Autodesk Fusion 360 part; units mm, degrees
(part 2 of 2)
sketch "Sketch2" plane through (0, 0, 25) normal (0, 0, 1) x (-1, 0, 0)
  spline S0 degree 3 poles (-93.3378, -102.7633) (-92.6534, -103.4892) (-92.135, -104.0698) (-92.1764, -104.0698) knots -1 -1 -1 -1 0 0 0 0
  spline S1 degree 3 poles (-92.1764, -104.0698) (-92.4046, -104.0698) (-94.6651, -102.2863) (-95.5154, -101.436) knots -1 -1 -1 -1 0 0 0 0
  spline S2 degree 3 poles (-95.5154, -101.436) (-96.0131, -100.9383) (-96.5938, -100.4406) (-96.8219, -100.3161) knots -1 -1 -1 -1 0 0 0 0
  spline S3 degree 3 poles (-96.8219, -100.3161) (-97.0293, -100.2125) (-97.1537, -100.0258) (-97.0915, -99.9014) knots -1 -1 -1 -1 0 0 0 0
  spline S4 degree 3 poles (-97.0915, -99.9014) (-97.0085, -99.7977) (-97.1537, -99.7147) (-97.3818, -99.7147) knots -1 -1 -1 -1 0 0 0 0
  spline S5 degree 3 poles (-97.3818, -99.7147) (-97.6307, -99.7147) (-97.921, -99.5281) (-98.0662, -99.3) knots -1 -1 -1 -1 0 0 0 0
  spline S6 degree 3 poles (-98.0662, -99.3) (-98.2114, -99.0718) (-98.4395, -98.8852) (-98.5847, -98.8852) knots -1 -1 -1 -1 0 0 0 0
  spline S7 degree 3 poles (-98.5847, -98.8852) (-98.7299, -98.8852) (-98.9165, -98.7608) (-98.9995, -98.5948) knots -1 -1 -1 -1 0 0 0 0
  spline S8 degree 3 poles (-98.9995, -98.5948) (-99.0824, -98.4289) (-99.4557, -97.9727) (-99.8083, -97.5786) knots -1 -1 -1 -1 0 0 0 0
  spline S9 degree 3 poles (-99.8083, -97.5786) (-101.0111, -96.2721) (-104.433, -91.6267) (-105.1588, -90.3201) knots -1 -1 -1 -1 0 0 0 0
  spline S10 degree 3 poles (-105.1588, -90.3201) (-106.258, -88.3707) (-108.1452, -83.663) (-108.7051, -81.5269) knots -1 -1 -1 -1 0 0 0 0
  spline S11 degree 3 poles (-108.7051, -81.5269) (-109.8043, -77.3377) (-110.2191, -72.4434) (-109.8665, -67.9639) knots -1 -1 -1 -1 0 0 0 0
  spline S12 degree 3 poles (-109.8665, -67.9639) (-109.5347, -63.7539) (-107.9171, -58.1545) (-106.1128, -54.8156) knots -1 -1 -1 -1 0 0 0 0
  spline S13 degree 3 poles (-106.1128, -54.8156) (-105.7395, -54.1312) (-105.2211, -53.2187) (-104.9929, -52.7624) knots -1 -1 -1 -1 0 0 0 0
  spline S14 degree 3 poles (-104.9929, -52.7624) (-104.7441, -52.3269) (-104.433, -51.9122) (-104.3086, -51.8707) knots -1 -1 -1 -1 0 0 0 0
  spline S15 degree 3 poles (-104.3086, -51.8707) (-104.1634, -51.8085) (-104.0389, -51.6011) (-104.0182, -51.4144) knots -1 -1 -1 -1 0 0 0 0
  spline S16 degree 3 poles (-104.0182, -51.4144) (-104.0182, -51.2278) (-103.956, -51.1863) (-103.8938, -51.3315) knots -1 -1 -1 -1 0 0 0 0
  spline S17 degree 3 poles (-103.8938, -51.3315) (-103.7693, -51.6633) (-103.1679, -51.0619) (-101.8407, -49.3198) knots -1 -1 -1 -1 0 0 0 0
  spline S18 degree 3 poles (-101.8407, -49.3198) (-99.6424, -46.3749) (-96.9256, -43.7411) (-93.6904, -41.3769) knots -1 -1 -1 -1 0 0 0 0
  spline S19 degree 3 poles (-93.6904, -41.3769) (-91.0151, -39.4275) (-86.5563, -36.9803) (-86.0171, -37.1877) knots -1 -1 -1 -1 0 0 0 0
  spline S20 degree 3 poles (-86.0171, -37.1877) (-85.8512, -37.2499) (-85.7682, -37.2499) (-85.8512, -37.167) knots -1 -1 -1 -1 0 0 0 0
  spline S21 degree 3 poles (-85.8512, -37.167) (-86.0585, -36.9596) (-83.3003, -35.7982) (-82.9478, -35.9434) knots -1 -1 -1 -1 0 0 0 0
  spline S22 degree 3 poles (-82.9478, -35.9434) (-82.7818, -35.9849) (-82.6989, -35.9641) (-82.7611, -35.8605) knots -1 -1 -1 -1 0 0 0 0
  spline S23 degree 3 poles (-82.7611, -35.8605) (-82.8233, -35.7568) (-82.6367, -35.6116) (-82.3049, -35.5494) knots -1 -1 -1 -1 0 0 0 0
  spline S24 degree 3 poles (-82.3049, -35.5494) (-81.9938, -35.4664) (-81.1435, -35.2383) (-80.3969, -35.0102) knots -1 -1 -1 -1 0 0 0 0
  spline S25 degree 3 poles (-80.3969, -35.0102) (-77.7009, -34.2428) (-77.2031, -34.1391) (-73.6983, -33.7451) knots -1 -1 -1 -1 0 0 0 0
  spline S26 degree 3 poles (-73.6983, -33.7451) (-69.8824, -33.3303) (-66.7924, -33.2474) (-66.2946, -33.5585) knots -1 -1 -1 -1 0 0 0 0
  spline S27 degree 3 poles (-66.2946, -33.5585) (-65.9628, -33.7659) (-66.1702, -33.8695) (-68.6796, -34.6991) knots -1 -1 -1 -1 0 0 0 0
  spline S28 degree 3 poles (-68.6796, -34.6991) (-70.8364, -35.4042) (-71.9355, -35.9641) (-74.4656, -37.6647) knots -1 -1 -1 -1 0 0 0 0
  spline S29 degree 3 poles (-74.4656, -37.6647) (-80.5421, -41.7502) (-87.054, -48.0963) (-90.2063, -53.0113) knots -1 -1 -1 -1 0 0 0 0
  spline S30 degree 3 poles (-90.2063, -53.0113) (-92.1142, -55.9562) (-93.4622, -59.1292) (-93.4622, -60.7053) knots -1 -1 -1 -1 0 0 0 0
  line L0 (-93.4622, -60.7053) -> (-93.483, -61.4519)
  line L1 (-93.483, -61.4519) -> (-94.0014, -60.8298)
  spline S31 degree 3 poles (-94.0014, -60.8298) (-95.6191, -58.8596) (-95.5154, -54.9815) (-93.6904, -49.4235) knots -1 -1 -1 -1 0 0 0 0
  spline S32 degree 3 poles (-93.6904, -49.4235) (-93.3585, -48.4073) (-93.1097, -47.5156) (-93.1512, -47.4741) knots -1 -1 -1 -1 0 0 0 0
  spline S33 degree 3 poles (-93.1512, -47.4741) (-93.3585, -47.2874) (-96.5108, -49.942) (-97.8588, -51.4144) knots -1 -1 -1 -1 0 0 0 0
  spline S34 degree 3 poles (-97.8588, -51.4144) (-101.8614, -55.811) (-103.6242, -59.3988) (-103.6242, -63.1525) knots -1 -1 -1 -1 0 0 0 0
  spline S35 degree 3 poles (-103.6242, -63.1525) (-103.6242, -66.1389) (-102.608, -69.0215) (-99.912, -73.584) knots -1 -1 -1 -1 0 0 0 0
  spline S36 degree 3 poles (-99.912, -73.584) (-97.8588, -77.0889) (-97.3404, -80.5522) (-98.2114, -84.9488) knots -1 -1 -1 -1 0 0 0 0
  spline S37 degree 3 poles (-98.2114, -84.9488) (-98.4603, -86.1309) (-98.7091, -87.9974) (-98.7713, -89.0965) knots -1 -1 -1 -1 0 0 0 0
  spline S38 degree 3 poles (-98.7713, -89.0965) (-99.0617, -93.8042) (-96.9878, -99.0511) (-93.3378, -102.7633) knots -1 -1 -1 -1 0 0 0 0
  spline S39 degree 3 poles (-53.9551, -98.2838) (-55.4691, -98.5119) (-56.6926, -98.346) (-58.1236, -97.6616) knots -1 -1 -1 -1 0 0 0 0
  spline S40 degree 3 poles (-58.1236, -97.6616) (-60.7989, -96.4173) (-63.1216, -93.1198) (-63.7023, -89.7394) knots -1 -1 -1 -1 0 0 0 0
  spline S41 degree 3 poles (-63.7023, -89.7394) (-63.8889, -88.7232) (-63.4327, -85.6954) (-62.9557, -84.7) knots -1 -1 -1 -1 0 0 0 0
  spline S42 degree 3 poles (-62.9557, -84.7) (-62.6031, -83.9534) (-62.5617, -83.5801) (-62.6861, -81.5477) knots -1 -1 -1 -1 0 0 0 0
  spline S43 degree 3 poles (-62.6861, -81.5477) (-62.8313, -78.9968) (-62.7691, -78.7272) (-61.5455, -77.5036) knots -1 -1 -1 -1 0 0 0 0
  spline S44 degree 3 poles (-61.5455, -77.5036) (-61.1307, -77.0889) (-60.5915, -76.4667) (-60.3219, -76.1142) knots -1 -1 -1 -1 0 0 0 0
  spline S45 degree 3 poles (-60.3219, -76.1142) (-59.5753, -75.098) (-57.5014, -74.7247) (-56.0497, -75.3261) knots -1 -1 -1 -1 0 0 0 0
  spline S46 degree 3 poles (-56.0497, -75.3261) (-55.6764, -75.4713) (-54.8884, -76.0312) (-54.287, -76.5704) knots -1 -1 -1 -1 0 0 0 0
  spline S47 degree 3 poles (-54.287, -76.5704) (-53.7063, -77.0889) (-52.856, -77.711) (-52.4412, -77.9184) knots -1 -1 -1 -1 0 0 0 0
  spline S48 degree 3 poles (-52.4412, -77.9184) (-51.1139, -78.6028) (-50.16, -79.7642) (-49.7037, -81.2366) knots -1 -1 -1 -1 0 0 0 0
  spline S49 degree 3 poles (-49.7037, -81.2366) (-49.206, -82.8127) (-49.206, -82.792) (-49.6, -82.6261) knots -1 -1 -1 -1 0 0 0 0
  spline S50 degree 3 poles (-49.6, -82.6261) (-49.7867, -82.5639) (-49.9111, -82.6261) (-49.9111, -82.8335) knots -1 -1 -1 -1 0 0 0 0
  spline S51 degree 3 poles (-49.9111, -82.8335) (-49.9111, -82.9994) (-49.9941, -83.0823) (-50.1185, -83.0201) knots -1 -1 -1 -1 0 0 0 0
  spline S52 degree 3 poles (-50.1185, -83.0201) (-50.2222, -82.9579) (-50.2637, -83.0201) (-50.2222, -83.1653) knots -1 -1 -1 -1 0 0 0 0
  spline S53 degree 3 poles (-50.2222, -83.1653) (-50.0977, -83.4764) (-51.2798, -84.7207) (-51.7776, -84.8244) knots -1 -1 -1 -1 0 0 0 0
  spline S54 degree 3 poles (-51.7776, -84.8244) (-52.5034, -84.9696) (-53.25, -86.3176) (-53.7685, -88.3914) knots -1 -1 -1 -1 0 0 0 0
  line L2 (-53.7685, -88.3914) -> (-54.1003, -89.7602)
  line L3 (-54.1003, -89.7602) -> (-54.9506, -89.0758)
  spline S55 degree 3 poles (-54.9506, -89.0758) (-56.3193, -87.9974) (-56.7548, -87.8315) (-58.6835, -87.7278) knots -1 -1 -1 -1 0 0 0 0
  spline S56 degree 3 poles (-58.6835, -87.7278) (-59.679, -87.6863) (-60.4878, -87.5619) (-60.4878, -87.4582) knots -1 -1 -1 -1 0 0 0 0
  spline S57 degree 3 poles (-60.4878, -87.4582) (-60.4878, -87.3545) (-60.633, -87.2715) (-60.8196, -87.2715) knots -1 -1 -1 -1 0 0 0 0
  spline S58 degree 3 poles (-60.8196, -87.2715) (-61.0063, -87.2715) (-61.11, -87.4167) (-61.0685, -87.6241) knots -1 -1 -1 -1 0 0 0 0
  spline S59 degree 3 poles (-61.0685, -87.6241) (-61.027, -87.8522) (-60.6537, -88.0389) (-59.8656, -88.184) knots -1 -1 -1 -1 0 0 0 0
  spline S60 degree 3 poles (-59.8656, -88.184) (-58.0821, -88.5573) (-56.7963, -89.3039) (-55.1165, -90.9423) knots -1 -1 -1 -1 0 0 0 0
  spline S61 degree 3 poles (-55.1165, -90.9423) (-54.287, -91.7718) (-53.5611, -92.4562) (-53.5196, -92.4562) knots -1 -1 -1 -1 0 0 0 0
  spline S62 degree 3 poles (-53.5196, -92.4562) (-53.4781, -92.4562) (-53.4367, -92.3318) (-53.4367, -92.1659) knots -1 -1 -1 -1 0 0 0 0
  spline S63 degree 3 poles (-53.4367, -92.1659) (-53.4367, -92.0207) (-52.8352, -90.6519) (-52.0887, -89.1588) knots -1 -1 -1 -1 0 0 0 0
  spline S64 degree 3 poles (-52.0887, -89.1588) (-50.8858, -86.7116) (-49.7867, -85.1977) (-49.2267, -85.1977) knots -1 -1 -1 -1 0 0 0 0
  spline S65 degree 3 poles (-49.2267, -85.1977) (-49.1438, -85.1977) (-48.9364, -85.5088) (-48.7705, -85.8821) knots -1 -1 -1 -1 0 0 0 0
  spline S66 degree 3 poles (-48.7705, -85.8821) (-47.9824, -87.6863) (-46.6137, -88.35) (-45.5145, -87.4789) knots -1 -1 -1 -1 0 0 0 0
  line L4 (-45.5145, -87.4789) -> (-44.996, -87.0849)
  line L5 (-44.996, -87.0849) -> (-44.8509, -88.2048)
  spline S67 degree 3 poles (-44.8509, -88.2048) (-44.7057, -89.4491) (-44.9546, -91.5644) (-45.5145, -93.8664) knots -1 -1 -1 -1 0 0 0 0
  spline S68 degree 3 poles (-45.5145, -93.8664) (-45.7841, -95.0693) (-46.0122, -95.5255) (-46.6137, -96.1062) knots -1 -1 -1 -1 0 0 0 0
  spline S69 degree 3 poles (-46.6137, -96.1062) (-47.4639, -96.9358) (-49.1645, -97.4957) (-50.3466, -97.309) knots -1 -1 -1 -1 0 0 0 0
  spline S70 degree 3 poles (-50.3466, -97.309) (-50.8858, -97.2261) (-51.3421, -97.309) (-52.0057, -97.6409) knots -1 -1 -1 -1 0 0 0 0
  spline S71 degree 3 poles (-52.0057, -97.6409) (-52.5034, -97.9105) (-53.3745, -98.1801) (-53.9551, -98.2838) knots -1 -1 -1 -1 0 0 0 0
  line L6 (-63.8475, -78.1673) -> (-64.0756, -78.9761)
  line L7 (-64.0756, -78.9761) -> (-64.5318, -78.5613)
  spline S72 degree 3 poles (-64.5318, -78.5613) (-64.7807, -78.3125) (-65.2577, -78.0636) (-65.5895, -77.9599) knots -1 -1 -1 -1 0 0 0 0
  spline S73 degree 3 poles (-65.5895, -77.9599) (-66.0458, -77.8355) (-66.2324, -77.6073) (-66.502, -76.8193) knots -1 -1 -1 -1 0 0 0 0
  spline S74 degree 3 poles (-66.502, -76.8193) (-66.6887, -76.2593) (-67.0205, -75.6579) (-67.2486, -75.4713) knots -1 -1 -1 -1 0 0 0 0
  spline S75 degree 3 poles (-67.2486, -75.4713) (-67.5182, -75.2431) (-67.7256, -74.7661) (-67.8085, -74.1025) knots -1 -1 -1 -1 0 0 0 0
  spline S76 degree 3 poles (-67.8085, -74.1025) (-68.1196, -71.9664) (-69.9239, -70.4732) (-72.2466, -70.4732) knots -1 -1 -1 -1 0 0 0 0
  spline S77 degree 3 poles (-72.2466, -70.4732) (-72.9102, -70.4732) (-74.1338, -70.6599) (-74.9426, -70.888) knots -1 -1 -1 -1 0 0 0 0
  spline S78 degree 3 poles (-74.9426, -70.888) (-76.8713, -71.4272) (-77.3691, -71.2613) (-77.7216, -70.017) knots -1 -1 -1 -1 0 0 0 0
  spline S79 degree 3 poles (-77.7216, -70.017) (-77.846, -69.5193) (-77.9083, -68.7105) (-77.846, -68.192) knots -1 -1 -1 -1 0 0 0 0
  spline S80 degree 3 poles (-77.846, -68.192) (-77.535, -65.7034) (-76.8713, -61.7838) (-76.6639, -61.2653) knots -1 -1 -1 -1 0 0 0 0
  spline S81 degree 3 poles (-76.6639, -61.2653) (-76.5395, -60.9335) (-75.8759, -60.0002) (-75.1915, -59.1914) knots -1 -1 -1 -1 0 0 0 0
  spline S82 degree 3 poles (-75.1915, -59.1914) (-74.4864, -58.3826) (-73.7813, -57.5323) (-73.5739, -57.3042) knots -1 -1 -1 -1 0 0 0 0
  spline S83 degree 3 poles (-73.5739, -57.3042) (-71.6867, -54.9815) (-67.0412, -49.5065) (-66.7924, -49.2991) knots -1 -1 -1 -1 0 0 0 0
  spline S84 degree 3 poles (-66.7924, -49.2991) (-66.3776, -48.9673) (-66.2531, -49.1539) (-65.631, -50.9789) knots -1 -1 -1 -1 0 0 0 0
  spline S85 degree 3 poles (-65.631, -50.9789) (-65.237, -52.161) (-65.1955, -52.721) (-65.237, -55.5414) knots -1 -1 -1 -1 0 0 0 0
  spline S86 degree 3 poles (-65.237, -55.5414) (-65.2784, -59.4403) (-65.0918, -60.7053) (-64.1378, -62.6963) knots -1 -1 -1 -1 0 0 0 0
  spline S87 degree 3 poles (-64.1378, -62.6963) (-63.5156, -63.9613) (-63.3912, -64.4383) (-63.412, -65.5374) knots -1 -1 -1 -1 0 0 0 0
  spline S88 degree 3 poles (-63.412, -65.5374) (-63.412, -67.0928) (-63.1631, -67.9846) (-62.4372, -69.0423) knots -1 -1 -1 -1 0 0 0 0
  spline S89 degree 3 poles (-62.4372, -69.0423) (-62.0017, -69.6644) (-60.9026, -70.6806) (-60.9026, -70.4318) knots -1 -1 -1 -1 0 0 0 0
  spline S90 degree 3 poles (-60.9026, -70.4318) (-60.9026, -70.3903) (-61.0477, -69.9133) (-61.2137, -69.3534) knots -1 -1 -1 -1 0 0 0 0
  spline S91 degree 3 poles (-61.2137, -69.3534) (-61.587, -68.1505) (-61.6284, -65.8278) (-61.2966, -64.8946) knots -1 -1 -1 -1 0 0 0 0
  spline S92 degree 3 poles (-61.2966, -64.8946) (-61.0892, -64.3139) (-61.1307, -64.065) (-61.4833, -63.2562) knots -1 -1 -1 -1 0 0 0 0
  spline S93 degree 3 poles (-61.4833, -63.2562) (-61.7321, -62.717) (-62.0847, -61.6801) (-62.2713, -60.9335) knots -1 -1 -1 -1 0 0 0 0
  spline S94 degree 3 poles (-62.2713, -60.9335) (-62.6446, -59.4196) (-62.9557, -56.1636) (-62.7276, -56.1636) knots -1 -1 -1 -1 0 0 0 0
  spline S95 degree 3 poles (-62.7276, -56.1636) (-62.5409, -56.1636) (-56.8171, -63.7747) (-55.4898, -65.8071) knots -1 -1 -1 -1 0 0 0 0
  spline S96 degree 3 poles (-55.4898, -65.8071) (-54.2247, -67.715) (-53.8722, -68.8971) (-53.6648, -71.7383) knots -1 -1 -1 -1 0 0 0 0
  spline S97 degree 3 poles (-53.6648, -71.7383) (-53.5404, -73.6877) (-53.4159, -74.2892) (-52.9597, -75.2017) knots -1 -1 -1 -1 0 0 0 0
  spline S98 degree 3 poles (-52.9597, -75.2017) (-52.6486, -75.7823) (-52.462, -76.2801) (-52.5656, -76.2801) knots -1 -1 -1 -1 0 0 0 0
  spline S99 degree 3 poles (-52.5656, -76.2801) (-52.6486, -76.2801) (-53.0634, -75.9482) (-53.4574, -75.5335) knots -1 -1 -1 -1 0 0 0 0
  spline S100 degree 3 poles (-53.4574, -75.5335) (-54.7017, -74.2477) (-55.3861, -73.9366) (-57.0452, -73.9366) knots -1 -1 -1 -1 0 0 0 0
  spline S101 degree 3 poles (-57.0452, -73.9366) (-57.854, -73.9366) (-58.9324, -73.9988) (-59.4509, -74.0818) knots -1 -1 -1 -1 0 0 0 0
  spline S102 degree 3 poles (-59.4509, -74.0818) (-60.3219, -74.2269) (-60.4878, -74.1855) (-61.6284, -73.4181) knots -1 -1 -1 -1 0 0 0 0
  spline S103 degree 3 poles (-61.6284, -73.4181) (-62.8105, -72.6508) (-63.6816, -71.8005) (-65.237, -69.8511) knots -1 -1 -1 -1 0 0 0 0
  spline S104 degree 3 poles (-65.237, -69.8511) (-66.7509, -67.9639) (-69.8617, -66.2218) (-71.4585, -66.367) knots -1 -1 -1 -1 0 0 0 0
  line L8 (-71.4585, -66.367) -> (-72.2051, -66.4292)
  line L9 (-72.2051, -66.4292) -> (-71.1889, -67.0306)
  spline S105 degree 3 poles (-71.1889, -67.0306) (-69.758, -67.8602) (-67.9952, -69.5193) (-66.9583, -70.971) knots -1 -1 -1 -1 0 0 0 0
  spline S106 degree 3 poles (-66.9583, -70.971) (-65.6725, -72.7752) (-65.3406, -73.1071) (-63.4327, -74.3514) knots -1 -1 -1 -1 0 0 0 0
  spline S107 degree 3 poles (-63.4327, -74.3514) (-62.2921, -75.0772) (-61.7736, -75.5542) (-61.8773, -75.7201) knots -1 -1 -1 -1 0 0 0 0
  spline S108 degree 3 poles (-61.8773, -75.7201) (-61.9602, -75.8653) (-62.375, -76.2801) (-62.8105, -76.6741) knots -1 -1 -1 -1 0 0 0 0
  spline S109 degree 3 poles (-62.8105, -76.6741) (-63.2668, -77.0681) (-63.7023, -77.711) (-63.8475, -78.1673) knots -1 -1 -1 -1 0 0 0 0
  spline S110 degree 3 poles (-44.5398, -70.8673) (-44.7057, -71.2198) (-44.8923, -71.5102) (-44.9753, -71.5102) knots -1 -1 -1 -1 0 0 0 0
  spline S111 degree 3 poles (-44.9753, -71.5102) (-45.2449, -71.5102) (-46.3233, -69.4985) (-47.0699, -67.5698) knots -1 -1 -1 -1 0 0 0 0
  spline S112 degree 3 poles (-47.0699, -67.5698) (-47.9824, -65.1642) (-48.7912, -62.4059) (-49.1023, -60.5602) knots -1 -1 -1 -1 0 0 0 0
  spline S113 degree 3 poles (-49.1023, -60.5602) (-49.6, -57.4909) (-50.1185, -55.3133) (-50.637, -53.986) knots -1 -1 -1 -1 0 0 0 0
  spline S114 degree 3 poles (-50.637, -53.986) (-50.948, -53.2394) (-51.1347, -52.5551) (-51.0725, -52.4928) knots -1 -1 -1 -1 0 0 0 0
  spline S115 degree 3 poles (-51.0725, -52.4928) (-50.8236, -52.2232) (-48.1898, -53.7579) (-47.0077, -54.8571) knots -1 -1 -1 -1 0 0 0 0
  spline S116 degree 3 poles (-47.0077, -54.8571) (-45.5767, -56.1636) (-44.7887, -57.4909) (-44.0421, -59.7306) knots -1 -1 -1 -1 0 0 0 0
  spline S117 degree 3 poles (-44.0421, -59.7306) (-43.254, -62.0534) (-42.9844, -64.3553) (-43.2747, -66.2011) knots -1 -1 -1 -1 0 0 0 0
  spline S118 degree 3 poles (-43.2747, -66.2011) (-43.5029, -67.7565) (-44.0628, -69.7681) (-44.5398, -70.8673) knots -1 -1 -1 -1 0 0 0 0
  spline S119 degree 3 poles (-69.4054, -110.167) (-72.0185, -110.2914) (-76.2906, -110.1048) (-77.6594, -109.7937) knots -1 -1 -1 -1 0 0 0 0
  spline S120 degree 3 poles (-77.6594, -109.7937) (-79.0074, -109.5034) (-79.5259, -109.2545) (-78.8, -109.2545) knots -1 -1 -1 -1 0 0 0 0
  spline S121 degree 3 poles (-78.8, -109.2545) (-76.8506, -109.2545) (-71.8733, -107.1184) (-69.4884, -105.2727) knots -1 -1 -1 -1 0 0 0 0
  spline S122 degree 3 poles (-69.4884, -105.2727) (-68.3477, -104.3809) (-67.7878, -104.0906) (-67.0205, -103.9661) knots -1 -1 -1 -1 0 0 0 0
  spline S123 degree 3 poles (-67.0205, -103.9661) (-63.9304, -103.5099) (-62.3958, -101.5605) (-62.6031, -98.3875) knots -1 -1 -1 -1 0 0 0 0
  line L10 (-62.6031, -98.3875) -> (-62.6861, -97.0394)
  line L11 (-62.6861, -97.0394) -> (-61.6284, -97.9519)
  spline S124 degree 3 poles (-61.6284, -97.9519) (-60.0523, -99.3) (-57.9992, -100.3369) (-56.7134, -100.4821) knots -1 -1 -1 -1 0 0 0 0
  spline S125 degree 3 poles (-56.7134, -100.4821) (-55.1995, -100.6272) (-52.3168, -100.0673) (-51.3421, -99.4036) knots -1 -1 -1 -1 0 0 0 0
  spline S126 degree 3 poles (-51.3421, -99.4036) (-50.8858, -99.1133) (-50.2429, -98.8852) (-49.8489, -98.8852) knots -1 -1 -1 -1 0 0 0 0
  spline S127 degree 3 poles (-49.8489, -98.8852) (-48.8534, -98.8852) (-46.9662, -98.346) (-45.7012, -97.7238) knots -1 -1 -1 -1 0 0 0 0
  spline S128 degree 3 poles (-45.7012, -97.7238) (-42.8807, -96.2929) (-42.2585, -95.1937) (-42.0304, -91.1082) knots -1 -1 -1 -1 0 0 0 0
  spline S129 degree 3 poles (-42.0304, -91.1082) (-41.9267, -89.6357) (-41.6571, -87.5204) (-41.4083, -86.442) knots -1 -1 -1 -1 0 0 0 0
  spline S130 degree 3 poles (-41.4083, -86.442) (-40.3506, -81.9625) (-41.0972, -77.2755) (-43.3784, -73.8951) knots -1 -1 -1 -1 0 0 0 0
  spline S131 degree 3 poles (-43.3784, -73.8951) (-43.6688, -73.4803) (-43.8347, -73.0448) (-43.7725, -72.9204) knots -1 -1 -1 -1 0 0 0 0
  spline S132 degree 3 poles (-43.7725, -72.9204) (-43.6895, -72.796) (-43.1503, -72.0286) (-42.5696, -71.2198) knots -1 -1 -1 -1 0 0 0 0
  spline S133 degree 3 poles (-42.5696, -71.2198) (-40.081, -67.7565) (-38.9818, -63.3392) (-39.8321, -60.2076) knots -1 -1 -1 -1 0 0 0 0
  spline S134 degree 3 poles (-39.8321, -60.2076) (-40.3713, -58.196) (-41.4497, -56.3502) (-42.9637, -54.8156) knots -1 -1 -1 -1 0 0 0 0
  spline S135 degree 3 poles (-42.9637, -54.8156) (-44.6227, -53.1565) (-46.0537, -52.3684) (-49.2267, -51.373) knots -1 -1 -1 -1 0 0 0 0
  spline S136 degree 3 poles (-49.2267, -51.373) (-50.3466, -51.0204) (-51.3835, -50.6678) (-51.5287, -50.5849) knots -1 -1 -1 -1 0 0 0 0
  spline S137 degree 3 poles (-51.5287, -50.5849) (-51.6946, -50.5227) (-52.2131, -49.5272) (-52.6901, -48.3866) knots -1 -1 -1 -1 0 0 0 0
  spline S138 degree 3 poles (-52.6901, -48.3866) (-54.8884, -43.2227) (-58.1443, -37.5403) (-60.0938, -35.4664) knots -1 -1 -1 -1 0 0 0 0
  spline S139 degree 3 poles (-60.0938, -35.4664) (-60.4463, -35.0931) (-60.6952, -34.7198) (-60.6122, -34.6576) knots -1 -1 -1 -1 0 0 0 0
  spline S140 degree 3 poles (-60.6122, -34.6576) (-60.4256, -34.471) (-56.4852, -36.1508) (-54.3284, -37.3329) knots -1 -1 -1 -1 0 0 0 0
  spline S141 degree 3 poles (-54.3284, -37.3329) (-49.7659, -39.8423) (-42.8392, -45.9809) (-39.8943, -50.1079) knots -1 -1 -1 -1 0 0 0 0
  spline S142 degree 3 poles (-39.8943, -50.1079) (-36.7835, -54.5045) (-34.9585, -59.5232) (-34.0046, -66.2218) knots -1 -1 -1 -1 0 0 0 0
  spline S143 degree 3 poles (-34.0046, -66.2218) (-33.569, -69.4156) (-33.7142, -75.1809) (-34.3156, -78.1051) knots -1 -1 -1 -1 0 0 0 0
  spline S144 degree 3 poles (-34.3156, -78.1051) (-35.1037, -81.838) (-36.6591, -86.5872) (-37.5509, -87.9974) knots -1 -1 -1 -1 0 0 0 0
  spline S145 degree 3 poles (-37.5509, -87.9974) (-37.696, -88.2255) (-38.1316, -88.9721) (-38.5048, -89.6565) knots -1 -1 -1 -1 0 0 0 0
  spline S146 degree 3 poles (-38.5048, -89.6565) (-38.8781, -90.3409) (-39.6662, -91.6474) (-40.2676, -92.5599) knots -1 -1 -1 -1 0 0 0 0
  spline S147 degree 3 poles (-40.2676, -92.5599) (-40.8691, -93.4724) (-41.3668, -94.3849) (-41.3875, -94.5923) knots -1 -1 -1 -1 0 0 0 0
  spline S148 degree 3 poles (-41.3875, -94.5923) (-41.4083, -94.7789) (-41.4497, -95.2352) (-41.4705, -95.567) knots -1 -1 -1 -1 0 0 0 0
  spline S149 degree 3 poles (-41.4705, -95.567) (-41.4912, -95.9196) (-41.6364, -96.1892) (-41.7816, -96.1892) knots -1 -1 -1 -1 0 0 0 0
  spline S150 degree 3 poles (-41.7816, -96.1892) (-41.9267, -96.1892) (-41.9889, -96.2929) (-41.906, -96.4173) knots -1 -1 -1 -1 0 0 0 0
  spline S151 degree 3 poles (-41.906, -96.4173) (-41.8438, -96.5417) (-42.1341, -97.0187) (-42.5696, -97.4542) knots -1 -1 -1 -1 0 0 0 0
  spline S152 degree 3 poles (-42.5696, -97.4542) (-43.2125, -98.0971) (-43.4821, -98.263) (-43.8969, -98.1801) knots -1 -1 -1 -1 0 0 0 0
  spline S153 degree 3 poles (-43.8969, -98.1801) (-44.1872, -98.1179) (-44.2909, -98.1179) (-44.1665, -98.1801) knots -1 -1 -1 -1 0 0 0 0
  spline S154 degree 3 poles (-44.1665, -98.1801) (-43.7517, -98.3667) (-43.8554, -98.6778) (-44.2909, -98.6778) knots -1 -1 -1 -1 0 0 0 0
  spline S155 degree 3 poles (-44.2909, -98.6778) (-44.5191, -98.6778) (-44.7679, -98.7608) (-44.8301, -98.8852) knots -1 -1 -1 -1 0 0 0 0
  spline S156 degree 3 poles (-44.8301, -98.8852) (-44.9131, -99.0096) (-44.8094, -99.0304) (-44.5813, -98.9474) knots -1 -1 -1 -1 0 0 0 0
  spline S157 degree 3 poles (-44.5813, -98.9474) (-44.2909, -98.8437) (-44.3117, -98.9267) (-44.7057, -99.3622) knots -1 -1 -1 -1 0 0 0 0
  spline S158 degree 3 poles (-44.7057, -99.3622) (-44.9753, -99.6733) (-45.2864, -99.8599) (-45.3901, -99.7977) knots -1 -1 -1 -1 0 0 0 0
  spline S159 degree 3 poles (-45.3901, -99.7977) (-45.4938, -99.7355) (-45.5352, -99.7562) (-45.5145, -99.8599) knots -1 -1 -1 -1 0 0 0 0
  spline S160 degree 3 poles (-45.5145, -99.8599) (-45.3279, -100.4198) (-49.1438, -103.4062) (-51.985, -104.9409) knots -1 -1 -1 -1 0 0 0 0
  spline S161 degree 3 poles (-51.985, -104.9409) (-52.5034, -105.2312) (-53.4367, -105.7289) (-54.0588, -106.0815) knots -1 -1 -1 -1 0 0 0 0
  spline S162 degree 3 poles (-54.0588, -106.0815) (-58.2066, -108.342) (-64.1585, -109.9181) (-69.4054, -110.167) knots -1 -1 -1 -1 0 0 0 0
  spline S163 degree 3 poles (-75.2952, -105.4386) (-80.5835, -107.1599) (-86.7429, -104.5261) (-91.1603, -98.6778) knots -1 -1 -1 -1 0 0 0 0
  spline S164 degree 3 poles (-91.1603, -98.6778) (-92.612, -96.7491) (-93.4622, -94.5508) (-94.0014, -91.4193) knots -1 -1 -1 -1 0 0 0 0
  spline S165 degree 3 poles (-94.0014, -91.4193) (-94.3125, -89.4491) (-94.3333, -88.9099) (-94.0844, -85.7161) knots -1 -1 -1 -1 0 0 0 0
  spline S166 degree 3 poles (-94.0844, -85.7161) (-93.9392, -83.7875) (-93.8355, -81.4855) (-93.8563, -80.6352) knots -1 -1 -1 -1 0 0 0 0
  spline S167 degree 3 poles (-93.8563, -80.6352) (-93.8978, -78.2502) (-94.831, -75.2846) (-95.9716, -73.8122) knots -1 -1 -1 -1 0 0 0 0
  spline S168 degree 3 poles (-95.9716, -73.8122) (-96.179, -73.5426) (-96.3034, -73.2522) (-96.2412, -73.1485) knots -1 -1 -1 -1 0 0 0 0
  spline S169 degree 3 poles (-96.2412, -73.1485) (-96.179, -73.0448) (-96.2412, -72.9619) (-96.3449, -72.9619) knots -1 -1 -1 -1 0 0 0 0
  spline S170 degree 3 poles (-96.3449, -72.9619) (-96.4693, -72.9619) (-96.573, -72.8167) (-96.573, -72.6301) knots -1 -1 -1 -1 0 0 0 0
  spline S171 degree 3 poles (-96.573, -72.6301) (-96.573, -72.4642) (-96.656, -72.3605) (-96.7389, -72.4227) knots -1 -1 -1 -1 0 0 0 0
  spline S172 degree 3 poles (-96.7389, -72.4227) (-96.9256, -72.5264) (-98.7506, -69.063) (-98.7506, -68.586) knots -1 -1 -1 -1 0 0 0 0
  spline S173 degree 3 poles (-98.7506, -68.586) (-98.7506, -68.3994) (-98.8543, -68.1298) (-98.9995, -67.9639) knots -1 -1 -1 -1 0 0 0 0
  spline S174 degree 3 poles (-98.9995, -67.9639) (-99.1239, -67.798) (-99.3105, -67.3832) (-99.3935, -67.0514) knots -1 -1 -1 -1 0 0 0 0
  spline S175 degree 3 poles (-99.3935, -67.0514) (-99.4764, -66.6988) (-99.6009, -66.3255) (-99.7046, -66.2218) knots -1 -1 -1 -1 0 0 0 0
  spline S176 degree 3 poles (-99.7046, -66.2218) (-99.7875, -66.0974) (-99.7875, -65.8693) (-99.6838, -65.7034) knots -1 -1 -1 -1 0 0 0 0
  spline S177 degree 3 poles (-99.6838, -65.7034) (-99.3728, -65.2264) (-99.435, -64.9982) (-99.7875, -65.2886) knots -1 -1 -1 -1 0 0 0 0
  spline S178 degree 3 poles (-99.7875, -65.2886) (-100.0364, -65.496) (-100.0779, -65.4338) (-100.0779, -64.936) knots -1 -1 -1 -1 0 0 0 0
  spline S179 degree 3 poles (-100.0779, -64.936) (-100.0779, -64.6249) (-100.1401, -63.7539) (-100.2438, -63.0073) knots -1 -1 -1 -1 0 0 0 0
  spline S180 degree 3 poles (-100.2438, -63.0073) (-100.4926, -61.1201) (-99.9534, -58.2997) (-99.1446, -57.0139) knots -1 -1 -1 -1 0 0 0 0
  spline S181 degree 3 poles (-99.1446, -57.0139) (-98.7921, -56.4747) (-96.9463, -54.6704) (-96.8426, -54.7741) knots -1 -1 -1 -1 0 0 0 0
  spline S182 degree 3 poles (-96.8426, -54.7741) (-96.8219, -54.8156) (-96.9463, -55.6659) (-97.133, -56.6821) knots -1 -1 -1 -1 0 0 0 0
  spline S183 degree 3 poles (-97.133, -56.6821) (-97.4026, -58.1752) (-97.4233, -58.8181) (-97.2574, -60.021) knots -1 -1 -1 -1 0 0 0 0
  spline S184 degree 3 poles (-97.2574, -60.021) (-96.9463, -62.1985) (-96.3242, -63.2769) (-94.3125, -65.1849) knots -1 -1 -1 -1 0 0 0 0
  spline S185 degree 3 poles (-94.3125, -65.1849) (-89.8537, -69.4363) (-89.3767, -69.9548) (-89.0034, -71.0954) knots -1 -1 -1 -1 0 0 0 0
  spline S186 degree 3 poles (-89.0034, -71.0954) (-88.485, -72.6508) (-88.6509, -75.2639) (-89.3975, -77.317) knots -1 -1 -1 -1 0 0 0 0
  spline S187 degree 3 poles (-89.3975, -77.317) (-89.7085, -78.1673) (-90.1441, -79.3701) (-90.3722, -79.9923) knots -1 -1 -1 -1 0 0 0 0
  spline S188 degree 3 poles (-90.3722, -79.9923) (-90.8699, -81.4232) (-90.8907, -83.9119) (-90.4137, -85.4051) knots -1 -1 -1 -1 0 0 0 0
  spline S189 degree 3 poles (-90.4137, -85.4051) (-89.7915, -87.313) (-87.925, -88.9306) (-85.2912, -89.8224) knots -1 -1 -1 -1 0 0 0 0
  spline S190 degree 3 poles (-85.2912, -89.8224) (-84.9387, -89.9261) (-82.5537, -90.0505) (-79.9821, -90.0713) knots -1 -1 -1 -1 0 0 0 0
  spline S191 degree 3 poles (-79.9821, -90.0713) (-76.021, -90.1127) (-75.0878, -90.175) (-73.8227, -90.5275) knots -1 -1 -1 -1 0 0 0 0
  spline S192 degree 3 poles (-73.8227, -90.5275) (-72.06, -91.0252) (-70.7327, -91.7718) (-69.7165, -92.8088) knots -1 -1 -1 -1 0 0 0 0
  spline S193 degree 3 poles (-69.7165, -92.8088) (-68.7625, -93.7835) (-67.5804, -96.1684) (-67.4145, -97.4542) knots -1 -1 -1 -1 0 0 0 0
  spline S194 degree 3 poles (-67.4145, -97.4542) (-67.3316, -98.0142) (-67.2071, -98.4704) (-67.1242, -98.4704) knots -1 -1 -1 -1 0 0 0 0
  spline S195 degree 3 poles (-67.1242, -98.4704) (-66.9583, -98.4704) (-65.631, -97.0602) (-64.8844, -96.0855) knots -1 -1 -1 -1 0 0 0 0
  line L12 (-64.8844, -96.0855) -> (-64.4074, -95.4633)
  line L13 (-64.4074, -95.4633) -> (-64.5111, -97.0187)
  spline S196 degree 3 poles (-64.5111, -97.0187) (-64.5526, -97.869) (-64.76, -99.0718) (-64.9674, -99.6525) knots -1 -1 -1 -1 0 0 0 0
  spline S197 degree 3 poles (-64.9674, -99.6525) (-65.2577, -100.5443) (-65.4651, -100.8346) (-66.1702, -101.2494) knots -1 -1 -1 -1 0 0 0 0
  spline S198 degree 3 poles (-66.1702, -101.2494) (-66.9997, -101.7264) (-67.2279, -101.7679) (-68.4929, -101.7886) knots -1 -1 -1 -1 0 0 0 0
  spline S199 degree 3 poles (-68.4929, -101.7886) (-68.9284, -101.8093) (-69.3225, -101.996) (-69.7372, -102.4315) knots -1 -1 -1 -1 0 0 0 0
  spline S200 degree 3 poles (-69.7372, -102.4315) (-70.5253, -103.261) (-73.4287, -104.8372) (-75.2952, -105.4386) knots -1 -1 -1 -1 0 0 0 0
  spline S201 degree 3 poles (-65.9213, -93.5554) (-66.0043, -93.742) (-66.1287, -93.9079) (-66.1702, -93.9079) knots -1 -1 -1 -1 0 0 0 0
  spline S202 degree 3 poles (-66.1702, -93.9079) (-66.2324, -93.9079) (-66.6057, -93.4102) (-67.0205, -92.788) knots -1 -1 -1 -1 0 0 0 0
  spline S203 degree 3 poles (-67.0205, -92.788) (-67.4352, -92.1659) (-68.2855, -91.2326) (-68.9492, -90.6934) knots -1 -1 -1 -1 0 0 0 0
  spline S204 degree 3 poles (-68.9492, -90.6934) (-70.0483, -89.7602) (-73.1176, -88.1011) (-73.6776, -88.1011) knots -1 -1 -1 -1 0 0 0 0
  spline S205 degree 3 poles (-73.6776, -88.1011) (-73.8227, -88.1011) (-74.0509, -87.9352) (-74.1546, -87.7485) knots -1 -1 -1 -1 0 0 0 0
  spline S206 degree 3 poles (-74.1546, -87.7485) (-74.279, -87.5411) (-74.3827, -87.4789) (-74.3827, -87.6034) knots -1 -1 -1 -1 0 0 0 0
  spline S207 degree 3 poles (-74.3827, -87.6034) (-74.3827, -87.7693) (-74.8389, -87.7278) (-75.8759, -87.4582) knots -1 -1 -1 -1 0 0 0 0
  spline S208 degree 3 poles (-75.8759, -87.4582) (-77.3483, -87.0642) (-79.2563, -86.7738) (-82.3256, -86.4835) knots -1 -1 -1 -1 0 0 0 0
  line L14 (-82.3256, -86.4835) -> (-83.9639, -86.3383)
  line L15 (-83.9639, -86.3383) -> (-83.5284, -85.7784)
  spline S209 degree 3 poles (-83.5284, -85.7784) (-83.2796, -85.488) (-83.0929, -85.1977) (-83.0929, -85.1355) knots -1 -1 -1 -1 0 0 0 0
  spline S210 degree 3 poles (-83.0929, -85.1355) (-83.0929, -85.0732) (-83.4455, -84.9696) (-83.8603, -84.8866) knots -1 -1 -1 -1 0 0 0 0
  spline S211 degree 3 poles (-83.8603, -84.8866) (-84.8764, -84.7) (-85.7889, -83.7252) (-85.7889, -82.8127) knots -1 -1 -1 -1 0 0 0 0
  spline S212 degree 3 poles (-85.7889, -82.8127) (-85.7889, -81.9832) (-84.9594, -81.1951) (-83.7151, -80.8218) knots -1 -1 -1 -1 0 0 0 0
  spline S213 degree 3 poles (-83.7151, -80.8218) (-83.2381, -80.6767) (-82.8855, -80.4485) (-82.8855, -80.2619) knots -1 -1 -1 -1 0 0 0 0
  spline S214 degree 3 poles (-82.8855, -80.2619) (-82.8855, -79.8471) (-85.4364, -80.013) (-86.3904, -80.49) knots -1 -1 -1 -1 0 0 0 0
  spline S215 degree 3 poles (-86.3904, -80.49) (-86.7844, -80.6767) (-87.137, -80.8011) (-87.1992, -80.7596) knots -1 -1 -1 -1 0 0 0 0
  spline S216 degree 3 poles (-87.1992, -80.7596) (-87.2406, -80.6974) (-86.9918, -80.013) (-86.6185, -79.2457) knots -1 -1 -1 -1 0 0 0 0
  spline S217 degree 3 poles (-86.6185, -79.2457) (-85.7267, -77.3792) (-85.1668, -75.5335) (-85.1668, -74.4758) knots -1 -1 -1 -1 0 0 0 0
  spline S218 degree 3 poles (-85.1668, -74.4758) (-85.1668, -72.4849) (-86.0793, -69.9548) (-87.5725, -67.7772) knots -1 -1 -1 -1 0 0 0 0
  line L16 (-87.5725, -67.7772) -> (-88.2776, -66.7403)
  line L17 (-88.2776, -66.7403) -> (-87.6969, -66.9684)
  spline S219 degree 3 poles (-87.6969, -66.9684) (-87.3858, -67.0928) (-86.4318, -67.1965) (-85.5816, -67.1965) knots -1 -1 -1 -1 0 0 0 0
  spline S220 degree 3 poles (-85.5816, -67.1965) (-83.5906, -67.2173) (-81.2679, -66.3463) (-79.671, -64.9775) knots -1 -1 -1 -1 0 0 0 0
  spline S221 degree 3 poles (-79.671, -64.9775) (-79.0696, -64.459) (-78.5304, -64.0443) (-78.4682, -64.0443) knots -1 -1 -1 -1 0 0 0 0
  spline S222 degree 3 poles (-78.4682, -64.0443) (-78.3438, -64.0443) (-78.3645, -64.2931) (-78.8622, -67.6321) knots -1 -1 -1 -1 0 0 0 0
  spline S223 degree 3 poles (-78.8622, -67.6321) (-79.3392, -70.8673) (-78.9452, -72.236) (-77.4105, -72.7545) knots -1 -1 -1 -1 0 0 0 0
  spline S224 degree 3 poles (-77.4105, -72.7545) (-76.8506, -72.9411) (-76.498, -72.8789) (-75.2952, -72.4227) knots -1 -1 -1 -1 0 0 0 0
  spline S225 degree 3 poles (-75.2952, -72.4227) (-71.8733, -71.1369) (-69.7372, -72.0909) (-69.0943, -75.1809) knots -1 -1 -1 -1 0 0 0 0
  spline S226 degree 3 poles (-69.0943, -75.1809) (-69.0321, -75.5542) (-68.6796, -76.1971) (-68.3477, -76.6119) knots -1 -1 -1 -1 0 0 0 0
  spline S227 degree 3 poles (-68.3477, -76.6119) (-68.0159, -77.0267) (-67.7463, -77.5451) (-67.7463, -77.7732) knots -1 -1 -1 -1 0 0 0 0
  spline S228 degree 3 poles (-67.7463, -77.7732) (-67.7463, -78.5198) (-67.1449, -79.3909) (-66.6264, -79.3909) knots -1 -1 -1 -1 0 0 0 0
  spline S229 degree 3 poles (-66.6264, -79.3909) (-65.7139, -79.3909) (-65.6102, -79.8471) (-66.1909, -81.2988) knots -1 -1 -1 -1 0 0 0 0
  spline S230 degree 3 poles (-66.1909, -81.2988) (-66.8338, -82.8542) (-67.2071, -85.3221) (-67.0412, -86.7531) knots -1 -1 -1 -1 0 0 0 0
  spline S231 degree 3 poles (-67.0412, -86.7531) (-66.979, -87.3338) (-66.6679, -88.4122) (-66.3776, -89.138) knots -1 -1 -1 -1 0 0 0 0
  spline S232 degree 3 poles (-66.3776, -89.138) (-65.8176, -90.486) (-65.5895, -92.7051) (-65.9213, -93.5554) knots -1 -1 -1 -1 0 0 0 0
  line L18 (-65.0088, -86.7116) -> (-65.3614, -88.1633)
  line L19 (-65.3614, -88.1633) -> (-65.5273, -87.2508)
  spline S233 degree 3 poles (-65.5273, -87.2508) (-65.7554, -86.0065) (-65.5273, -84.3267) (-64.9259, -82.709) knots -1 -1 -1 -1 0 0 0 0
  spline S234 degree 3 poles (-64.9259, -82.709) (-64.3659, -81.2781) (-63.9926, -80.8426) (-63.7645, -81.4232) knots -1 -1 -1 -1 0 0 0 0
  spline S235 degree 3 poles (-63.7645, -81.4232) (-63.4949, -82.1284) (-63.5986, -82.9994) (-64.1378, -84.1193) knots -1 -1 -1 -1 0 0 0 0
  spline S236 degree 3 poles (-64.1378, -84.1193) (-64.4281, -84.7414) (-64.8222, -85.9028) (-65.0088, -86.7116) knots -1 -1 -1 -1 0 0 0 0
  spline S237 degree 3 poles (-42.9222, -83.6008) (-42.86, -85.6125) (-42.86, -87.2715) (-42.9429, -87.2715) knots -1 -1 -1 -1 0 0 0 0
  spline S238 degree 3 poles (-42.9429, -87.2715) (-43.0051, -87.2715) (-43.3784, -86.6494) (-43.731, -85.8821) knots -1 -1 -1 -1 0 0 0 0
  spline S239 degree 3 poles (-43.731, -85.8821) (-44.3531, -84.5963) (-44.4154, -84.2852) (-44.4154, -82.5017) knots -1 -1 -1 -1 0 0 0 0
  spline S240 degree 3 poles (-44.4154, -82.5017) (-44.4154, -80.7804) (-44.4983, -80.3656) (-45.0168, -79.2457) knots -1 -1 -1 -1 0 0 0 0
  spline S241 degree 3 poles (-45.0168, -79.2457) (-45.3279, -78.5406) (-45.7841, -77.794) (-46.0122, -77.5866) knots -1 -1 -1 -1 0 0 0 0
  spline S242 degree 3 poles (-46.0122, -77.5866) (-46.427, -77.2133) (-46.427, -77.234) (-46.2818, -78.9761) knots -1 -1 -1 -1 0 0 0 0
  spline S243 degree 3 poles (-46.2818, -78.9761) (-46.1989, -79.9508) (-46.0744, -81.2781) (-45.9915, -81.921) knots -1 -1 -1 -1 0 0 0 0
  spline S244 degree 3 poles (-45.9915, -81.921) (-45.8048, -83.3934) (-46.1574, -85.5917) (-46.6344, -85.9028) knots -1 -1 -1 -1 0 0 0 0
  spline S245 degree 3 poles (-46.6344, -85.9028) (-47.2773, -86.2968) (-47.6298, -85.6954) (-47.6298, -84.2644) knots -1 -1 -1 -1 0 0 0 0
  spline S246 degree 3 poles (-47.6298, -84.2644) (-47.6298, -82.5224) (-48.1068, -81.1329) (-49.4341, -79.1213) knots -1 -1 -1 -1 0 0 0 0
  spline S247 degree 3 poles (-49.4341, -79.1213) (-51.508, -75.9275) (-51.6117, -75.5957) (-51.7568, -72.0286) knots -1 -1 -1 -1 0 0 0 0
  spline S248 degree 3 poles (-51.7568, -72.0286) (-51.8813, -69.063) (-51.9227, -68.8349) (-52.5449, -67.5698) knots -1 -1 -1 -1 0 0 0 0
  spline S249 degree 3 poles (-52.5449, -67.5698) (-53.1463, -66.3463) (-54.4943, -64.5627) (-56.8378, -61.9289) knots -1 -1 -1 -1 0 0 0 0
  spline S250 degree 3 poles (-56.8378, -61.9289) (-59.285, -59.1707) (-60.6745, -57.0346) (-62.6654, -52.9491) knots -1 -1 -1 -1 0 0 0 0
  spline S251 degree 3 poles (-62.6654, -52.9491) (-64.2415, -49.7346) (-64.9881, -47.5156) (-65.5895, -44.3218) knots -1 -1 -1 -1 0 0 0 0
  spline S252 degree 3 poles (-65.5895, -44.3218) (-65.7762, -43.3056) (-66.0043, -42.4761) (-66.108, -42.4761) knots -1 -1 -1 -1 0 0 0 0
  spline S253 degree 3 poles (-66.108, -42.4761) (-66.2117, -42.4761) (-66.4813, -42.8701) (-66.7509, -43.3678) knots -1 -1 -1 -1 0 0 0 0
  spline S254 degree 3 poles (-66.7509, -43.3678) (-67.1034, -44.0522) (-67.1864, -44.5707) (-67.1656, -45.732) knots -1 -1 -1 -1 0 0 0 0
  line L20 (-67.1656, -45.732) -> (-67.1449, -47.246)
  line L21 (-67.1449, -47.246) -> (-68.4307, -48.8428)
  spline S255 degree 3 poles (-68.4307, -48.8428) (-69.1566, -49.7346) (-70.9816, -52.1403) (-72.5162, -54.1934) knots -1 -1 -1 -1 0 0 0 0
  spline S256 degree 3 poles (-72.5162, -54.1934) (-77.7009, -61.1201) (-80.1895, -63.9821) (-81.7034, -64.7286) knots -1 -1 -1 -1 0 0 0 0
  spline S257 degree 3 poles (-81.7034, -64.7286) (-84.6691, -66.2426) (-88.402, -65.7241) (-90.2478, -63.5673) knots -1 -1 -1 -1 0 0 0 0
  spline S258 degree 3 poles (-90.2478, -63.5673) (-90.8492, -62.8622) (-90.9736, -62.5718) (-90.9736, -61.763) knots -1 -1 -1 -1 0 0 0 0
  spline S259 degree 3 poles (-90.9736, -61.763) (-90.9736, -59.938) (-89.9159, -56.8894) (-88.879, -55.6451) knots -1 -1 -1 -1 0 0 0 0
  spline S260 degree 3 poles (-88.879, -55.6451) (-84.752, -50.7923) (-79.0696, -44.9025) (-78.2816, -44.6329) knots -1 -1 -1 -1 0 0 0 0
  spline S261 degree 3 poles (-78.2816, -44.6329) (-78.0742, -44.5707) (-77.9083, -44.4463) (-77.9083, -44.3426) knots -1 -1 -1 -1 0 0 0 0
  spline S262 degree 3 poles (-77.9083, -44.3426) (-77.9083, -44.1144) (-74.6108, -41.6465) (-74.2997, -41.6465) knots -1 -1 -1 -1 0 0 0 0
  spline S263 degree 3 poles (-74.2997, -41.6465) (-74.1753, -41.6465) (-73.9679, -41.4806) (-73.8435, -41.2732) knots -1 -1 -1 -1 0 0 0 0
  spline S264 degree 3 poles (-73.8435, -41.2732) (-73.3872, -40.5474) (-68.2648, -37.6855) (-66.2117, -37.0011) knots -1 -1 -1 -1 0 0 0 0
  spline S265 degree 3 poles (-66.2117, -37.0011) (-64.9051, -36.5656) (-63.5156, -36.6278) (-62.6861, -37.1877) knots -1 -1 -1 -1 0 0 0 0
  spline S266 degree 3 poles (-62.6861, -37.1877) (-61.1514, -38.2247) (-58.3102, -42.5176) (-55.6557, -47.8681) knots -1 -1 -1 -1 0 0 0 0
  spline S267 degree 3 poles (-55.6557, -47.8681) (-53.4159, -52.3684) (-52.2338, -55.6659) (-50.8443, -61.3897) knots -1 -1 -1 -1 0 0 0 0
  spline S268 degree 3 poles (-50.8443, -61.3897) (-49.1852, -68.192) (-48.3557, -70.3281) (-46.6137, -72.2568) knots -1 -1 -1 -1 0 0 0 0
  spline S269 degree 3 poles (-46.6137, -72.2568) (-45.7634, -73.1693) (-45.3901, -73.7914) (-44.1872, -76.0934) knots -1 -1 -1 -1 0 0 0 0
  spline S270 degree 3 poles (-44.1872, -76.0934) (-43.4199, -77.5451) (-43.0259, -79.9093) (-42.9222, -83.6008) knots -1 -1 -1 -1 0 0 0 0
  circle A0 centre (-71.2861, -71.324) radius 43.4137
  line L22 (-45.4271, -30.1036) -> (-103.5259, -30.1036)
  line L23 (-103.5259, -30.1036) -> (-103.5259, -20.3009)
  line L24 (-103.5259, -20.3009) -> (-45.4271, -20.3009)
  line L25 (-45.4271, -20.3009) -> (-45.4271, -30.1036)
  constraint horizontal L22
  constraint vertical L23
  constraint horizontal L24
  constraint vertical L25
extrude "Extrude2" cut sketch "Sketch2" against normal blind 27 contours A0 L22 picked at (-70.3628, -29.402)
